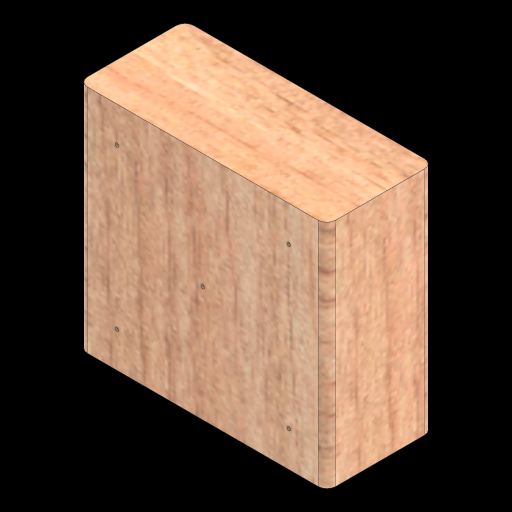
# Autodesk Inventor part: Square
Saved by Autodesk Inventor 2024.2 (Build 282272000, 272)
## iProperties
Created: 2025-06-28
Part Number: Square
Material: Wood (Birch)
Document SubType Name: Modeling
Designer: Bryan
Density: 0.55 g/cm^3
Appearance: Birch - Natural Polished
Mass: 2263.95 g
Surface Area: 3130.66 cm^2
Volume: 4116.28 cm^3
Author: Bryan
Autodesk Inventor part; units mm, degrees
ref_plane "YZ Plane" through (0, 0, 0) normal (1, 0, 0) x (0, 1, 0)
ref_plane "XZ Plane" through (0, 0, 0) normal (0, 1, 0) x (-1, 0, 0)
ref_plane "XY Plane" through (0, 0, 0) normal (0, 0, 1) x (1, 0, 0)
sketch "Sketch1" plane through (0, 0, 0) normal (0, 1, 0) x (-1, 0, 0)
  line L0 (3.175, 0) -> (85.725, 0)
  line L1 (88.9, -3.175) -> (88.9, -34.925)
  line L2 (85.725, -38.1) -> (3.175, -38.1)
  line L3 (0, -34.925) -> (0, -3.175)
  arc A0 (88.9, -3.175) -> (85.725, 0) centre (85.725, -3.175) ccw
  arc A1 (85.725, -38.1) -> (88.9, -34.925) centre (85.725, -34.925) ccw
  arc A2 (0, -34.925) -> (3.175, -38.1) centre (3.175, -34.925) ccw
  arc A3 (3.175, 0) -> (0, -3.175) centre (3.175, -3.175) ccw
  point P0 (0, 0)
  point P1 (88.9, -38.1)
  point P2 (88.9, 0)
  point P3 (0, -38.1)
  dimension "d0" = 88.9
  dimension "d1" = 38.1
  dimension "d2" = 3.175
  constraints: 8 end point, 8 point on circle, 8 point on line, 8 tangent, 4 centre point, 3 equal radius, 2 parallel, 1 horizontal, 1 perpendicular
  measures "d0" distance of point (88.9, -38.1) point (0, -38.1)
  measures "d1" distance of point (88.9, 0) point (88.9, -38.1)
  measures "d2" radius of A0
extrude "Extrusion1" add sketch "Sketch1" along normal blind 82.55
sketch "Sketch2" plane through (-3.175, 0, -38.1) normal (0, 0, -1) x (-1, 0, 0)
  line L0 (0, 0) -> (82.55, 0) construction
  line L1 (82.55, 0) -> (82.55, 82.55) construction
  line L2 (0, 82.55) -> (82.55, 82.55) construction
  line L3 (0, 0) -> (0, 82.55) construction
  line L4 (60.325, 82.55) -> (60.325, 61.9125) construction
  line L5 (60.325, 61.9125) -> (60.325, 41.275) construction
  line L6 (60.325, 41.275) -> (60.325, 20.6375) construction
  line L7 (60.325, 20.6375) -> (60.325, 0) construction
  circle A0 centre (60.325, 88.1126) radius 1.5875
  circle A1 centre (60.325, 35.7124) radius 1.5875
  circle A2 centre (60.325, 67.4751) radius 1.5875
  circle A3 centre (60.325, 15.0749) radius 1.5875
  circle A4 centre (60.325, 46.8376) radius 1.5875
  circle A5 centre (60.325, -5.5626) radius 1.5875
  line L8 (85.725, 0) -> (85.725, 82.55) projected
  line L9 (60.325, 61.9125) -> (22.225, 61.9125) construction
  circle A6 centre (22.225, 61.9125) radius 1.5875
  line L10 (60.325, 41.275) -> (22.225, 41.275) construction
  circle A7 centre (22.225, 41.275) radius 1.5875
  line L11 (60.325, 20.6375) -> (22.225, 20.6375) construction
  circle A8 centre (22.225, 20.6375) radius 1.5875
  point P0 (-3.175, 0)
  point P1 (85.725, 41.275)
  dimension "d5" = 3.175
  dimension "d6" = 26.2001
  dimension "d7" = 26.2001
  dimension "d8" = 3.175
  dimension "d9" = 26.2001
  dimension "d10" = 26.2001
  dimension "d11" = 3.175
  dimension "d12" = 26.2001
  dimension "d13" = 26.2001
  dimension "d16" = 25.4
  dimension "d17" = 38.1
  dimension "d18" = 38.1
  dimension "d19" = 38.1
  constraints: 14 end point, 12 coincident, 9 centre point, 6 equal radius, 5 point on line, 4 vertical alignment, 3 collinear, 3 horizontal, 2 vertical, 1 horizontal alignment, 1 midpoint
  measures "d5" diameter of A0
  measures "d6" distance of L9.start A0.centre
  measures "d7" distance of A1.centre L9.start
  measures "d8" diameter of A2
  measures "d9" distance of point (60.325, 41.275) A2.centre
  measures "d10" distance of A3.centre point (60.325, 41.275)
  measures "d11" diameter of A4
  measures "d12" distance of point (60.325, 20.637) A4.centre
  measures "d13" distance of A5.centre point (60.325, 20.637)
  measures "d16" distance between parallel lines of L8 L4
  measures "d17" distance of L9.start L9.end
  measures "d18" distance of L10.start L10.end
  measures "d19" distance of L11.start L11.end
extrude "Extrusion2" [suppressed]
sketch "Sketch3" plane through (-85.725, 0, 0) normal (0, 0, 1) x (1, 0, 0)
  line L0 (0, 0) -> (-3.175, 0) construction
  line L1 (85.725, 82.55) -> (82.55, 82.55) construction
  line L2 (-3.175, 0) -> (85.725, 0) construction
  line L3 (85.725, 0) -> (85.725, 82.55) construction
  line L4 (85.725, 82.55) -> (-3.175, 82.55) construction
  line L5 (-3.175, 82.55) -> (-3.175, 0) construction
  line L6 (-3.175, 82.55) -> (85.725, 82.55) construction
  line L7 (85.725, 82.55) -> (85.725, 0) construction
  line L8 (85.725, 0) -> (-3.175, 0) construction
  line L9 (-3.175, 0) -> (-3.175, 82.55) construction
  line L10 (-3.175, 82.55) -> (85.725, 0) construction
  line L11 (85.725, 82.55) -> (-3.175, 0) construction
  line L12 (0, 82.55) -> (82.55, 82.55) projected
  circle A0 centre (10.5019, 12.7) radius 0.635
  circle A1 centre (10.5019, 69.85) radius 0.635
  circle A2 centre (72.0481, 69.85) radius 0.635
  circle A3 centre (72.0481, 12.7) radius 0.635
  line L13 (72.0481, 12.7) -> (72.0481, 69.85) construction
  line L14 (10.5019, 12.7) -> (10.5019, 69.85) construction
  circle A4 centre (41.275, 41.275) radius 0.635
  dimension "d20" = 1.27
  dimension "d21" = 12.7
  constraints: 24 end point, 5 centre point, 5 point on line, 4 equal radius, 4 parallel, 2 equal length, 2 horizontal, 2 midpoint, 2 perpendicular, 2 vertical, 1 coincident
  measures "d20" diameter of A0
  measures "d21" distance from line of L8 L14.start
extrude "Extrusion3" cut sketch "Sketch3" against normal through all
equation "\"d7\" = d6"
equation "\"d10\" = d9"
equation "\"d13\" = d12"
body "Solid1"
